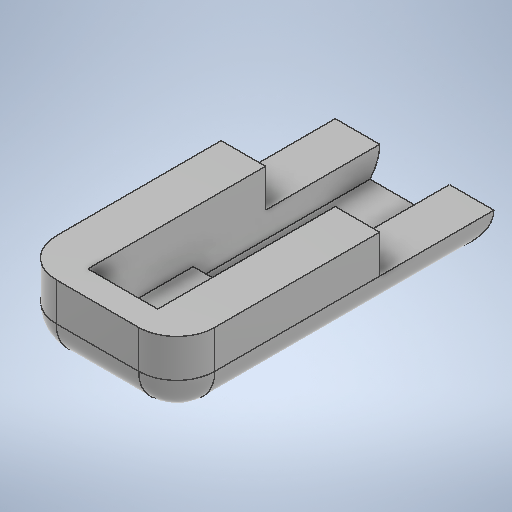
# Autodesk Inventor part: pressure_plate
Saved by Autodesk Inventor 2025 (Build 290162000, 162)
## iProperties
Created: 2025-09-02
Part Number: pressure_plate
Material: ABS プラスチック
Document SubType Name: Modeling
Designer: sooo1
Density: 1.06 g/cm^3
Appearance: 滑らか - 標準の灰色
Author: sooo1
Autodesk Inventor part; units mm, degrees
ref_plane "YZ Plane" through (0, 0, 0) normal (1, 0, 0) x (0, 1, 0)
ref_plane "XZ Plane" through (0, 0, 0) normal (0, 1, 0) x (-1, 0, 0)
ref_plane "XY Plane" through (0, 0, 0) normal (0, 0, 1) x (1, 0, 0)
sketch "スケッチ1" plane through (0, 0, 0) normal (0, 1, 0) x (-1, 0, 0)
  line L0 (12.5, 22.5) -> (-12.5, 22.5)
  line L1 (-12.5, 22.5) -> (-12.5, -22.5)
  line L2 (-12.5, -22.5) -> (12.5, -22.5)
  line L3 (12.5, -22.5) -> (12.5, 22.5)
  line L4 (12.5, 22.5) -> (-12.5, -22.5) construction
  line L5 (-12.5, 22.5) -> (12.5, -22.5) construction
  line L6 (12.5, 22.5) -> (12.5, 27.5)
  line L7 (12.5, 27.5) -> (-12.5, 27.5)
  line L8 (-12.5, 27.5) -> (-12.5, 22.5)
  point P0 (0, 0)
  dimension "d0" = 45
  dimension "d2" = 25
  dimension "d3" = 5
  constraints: 18 end point, 3 perpendicular, 2 midpoint, 2 parallel, 1 horizontal, 1 vertical
  measures "d0" distance of L2.end L0.start
  measures "d2" distance of L1.end L2.end
  measures "d3" distance between parallel lines of L0 L7
extrude "押し出し1" add sketch "スケッチ1" along normal blind 2
sketch "スケッチ2" plane through (0, 2, 0) normal (0, 1, 0) x (1, 0, 0)
  line L0 (-12.5, -27.5) -> (12.5, -27.5) construction
  line L1 (12.5, -27.5) -> (12.5, 22.5) construction
  line L2 (12.5, 22.5) -> (-12.5, 22.5) construction
  line L3 (-12.5, 22.5) -> (-12.5, -27.5) construction
  line L4 (0, 32.5) -> (0, -37.5) construction
  line L5 (-12.5, -27.5) -> (12.5, -27.5)
  line L6 (12.5, -27.5) -> (12.5, 22.5)
  line L7 (12.5, 22.5) -> (-12.5, 22.5)
  line L8 (-12.5, 22.5) -> (-12.5, -27.5)
  line L9 (-12.5, 22.5) -> (-12.5, -27.5) projected
  line L10 (12.5, 22.5) -> (-12.5, 22.5) projected
  point P0 (0, 0)
  point P1 (0, -27.5)
  constraints: 8 end point, 2 collinear, 2 parallel, 2 point on line, 1 horizontal, 1 midpoint, 1 perpendicular
extrude "押し出し2" add sketch "スケッチ2" along normal blind 2
sketch "スケッチ3" plane through (0, 4, 0) normal (0, 1, 0) x (1, 0, 0)
  line L0 (-12.5, 22.5) -> (-12.5, -2) construction
  line L1 (-12.5, -2) -> (12.5, -2) construction
  line L2 (12.5, -2) -> (12.5, 22.5) construction
  line L3 (12.5, 22.5) -> (-12.5, 22.5) construction
  line L4 (-12.5, 22.5) -> (-12.5, -2) construction
  line L5 (-12.5, -27.5) -> (12.5, -27.5)
  line L6 (12.5, -27.5) -> (12.5, 22.5)
  line L7 (12.5, 22.5) -> (-12.5, 22.5)
  line L8 (-12.5, 22.5) -> (-12.5, -27.5)
  line L9 (-12.5, -27.5) -> (12.5, -27.5) construction
  point P0 (0, 0)
  constraints: 8 end point, 2 parallel, 1 collinear, 1 horizontal, 1 perpendicular
extrude "押し出し3" add sketch "スケッチ3" along normal blind 8
sketch "スケッチ4" plane through (0, 12, 0) normal (0, 1, 0) x (1, 0, 0)
  line L0 (12.5, -2) -> (12.5, 22.5) construction
  line L1 (-5.5, 22.5) -> (5.5, 22.5)
  line L2 (5.5, 22.5) -> (5.5, -23.5)
  line L3 (5.5, -23.5) -> (-5.5, -23.5)
  line L4 (-5.5, -23.5) -> (-5.5, 22.5)
  line L5 (0, 32.5) -> (0, -37.5) construction
  circle A0 centre (0, -18.4) radius 1.5
  circle A1 centre (0, -11) radius 1.5
  line L6 (-17.5, 0) -> (17.5, 0) construction
  line L7 (-5.5, -6.9) -> (5.5, -6.9)
  line L8 (12.5, -27.5) -> (12.5, 22.5) construction
  line L9 (12.5, 22.5) -> (-12.5, 22.5) construction
  line L10 (-12.5, 22.5) -> (-12.5, -27.5) construction
  line L11 (-12.5, -27.5) -> (12.5, -27.5) construction
  line L12 (12.5, 22.5) -> (-12.5, 22.5) projected
  point P0 (0, 0)
  point P1 (0, -23.5)
  dimension "d14" = 11
  dimension "d15" = 3
  dimension "d16" = 7.4
  dimension "d17" = 22
  dimension "d24" = 16.6
  dimension "d27" = 46
  constraints: 10 end point, 5 point on line, 2 centre point, 2 parallel, 2 perpendicular, 1 collinear, 1 equal radius, 1 horizontal, 1 midpoint
  measures "d14" distance of L2.end L3.end
  measures "d15" diameter of A1
  measures "d16" distance of A0.centre A1.centre
  measures "d17" diameter of A1.centre L6
  measures "d24" distance between parallel lines of L3 L7
  measures "d27" distance of L3.end L1.start
extrude "押し出し4" cut sketch "スケッチ4" against normal blind 8 contours L1 L2 L7 L4 | L7 L2 L3 L4 | A0 | A1
extrude "押し出し5" cut sketch "スケッチ4" against normal through all contours A0 | A1
extrude "押し出し6" cut sketch "スケッチ4" against normal blind 10 contours L1 L2 L7 L4
sketch "スケッチ5" plane through (0, 0, 0) normal (0, -1, 0) x (1, 0, 0)
  circle A0 centre (0, 18.4) radius 1.5 construction
  circle A1 centre (0, 11) radius 1.5 construction
  circle A2 centre (0, 18.4) radius 2.75
  circle A3 centre (0, 11) radius 2.75
  point P0 (0, 0)
  dimension "d28" = 5.5
  constraints: 2 centre point, 2 coincident, 1 equal radius
  measures "d28" diameter of A2
extrude "押し出し7" cut sketch "スケッチ5" against normal blind 2.5
fillet "フィレット1" radius 6 6 edges at (12.5, 0, 2.5) (-12.5, 0, 2.5) (0, 0, 27.5) (12.5, 6, 27.5) (-12.5, 6, 27.5) (0, 0, -22.5)
sketch "スケッチ6" plane through (0, 0, 0) normal (1, 0, 0) x (0, 1, 0)
  line L0 (12, 23.5) -> (12, -22.5) construction
  line L1 (12, -22.5) -> (2, -22.5) construction
  line L2 (12, -22.5) -> (6, -22.5)
  line L3 (6, -22.5) -> (6, -4.5)
  line L4 (6, -4.5) -> (12, -4.5)
  line L5 (12, -4.5) -> (12, -22.5)
  point P0 (0, 0)
  dimension "d32" = 6
  dimension "d33" = 18
  constraints: 8 end point, 2 parallel, 1 horizontal, 1 perpendicular
  measures "d32" distance of L3.end L4.end
  measures "d33" distance of L2.end L3.end
extrude "押し出し8" cut sketch "スケッチ6" along normal through all both and the other way through all
sketch "スケッチ7" plane through (0, 12, 0) normal (0, 1, 0) x (1, 0, 0)
  line L0 (5.5, -6.9) -> (-5.5, -6.9) projected
  line L1 (-28.6346, -6.9) -> (35.9523, -6.9)
  line L2 (35.9523, -6.9) -> (35.9523, 63.9707)
  line L3 (35.9523, 63.9707) -> (-28.6346, 63.9707)
  line L4 (-28.6346, 63.9707) -> (-28.6346, -6.9)
  point P0 (0, 0)
  constraints: 8 end point, 2 parallel, 1 collinear, 1 horizontal, 1 perpendicular
